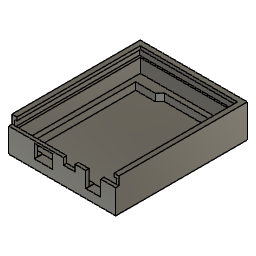
boitier VF Soufiani_Younousse (Autodesk Fusion 360 design; units mm, degrees)
Autodesk Fusion 360 part; units mm, degrees
note: some values were not read from the file. Set by a fixed rule: which sketch regions a step uses.
sketch "Esquisse1" plane through (0, 0, 0) normal (0, 0, 1) x (1, 0, 0)
  line L0 (0, 0) -> (53.1, 0)
  line L1 (53.1, 0) -> (53.1, 66.2)
  line L2 (0, 66.2) -> (0, 0)
  line L3 (40.9, 0) -> (49.9, 0)
  line L4 (49.9, 0) -> (49.9, -5.2)
  line L5 (49.9, -5.2) -> (40.9, -5.2)
  line L6 (40.9, -5.2) -> (40.9, 0)
  line L7 (11.5, 0) -> (18.8, 0)
  line L8 (18.8, 0) -> (18.8, -1.2)
  line L9 (18.8, -1.2) -> (11.5, -1.2)
  line L10 (11.5, -1.2) -> (11.5, 0)
  line L11 (53.1, 66.2) -> (50.8, 66.2) construction
  line L12 (50.8, 66.2) -> (48.7068, 69)
  line L13 (48.7068, 69) -> (14.6068, 69)
  line L14 (12.1, 66.2) -> (14.6068, 69)
  line L15 (53.1, 66.2) -> (50.8, 66.2)
  line L16 (12.1, 66.2) -> (0, 66.2)
  line L17 (40.9, 0) -> (49.9, 0)
  line L18 (11.5, 0) -> (18.8, 0)
  line L19 (0, 33.1) -> (53.1, 33.1) construction
  line L20 (26.55, 0) -> (26.55, 33.1) construction
  line L21 (0, 66.2) -> (0, 68.7) construction
  line L22 (0, 68.7) -> (53.1, 68.7) construction
  line L23 (53.1, 68.7) -> (53.1, 66.2) construction
  line L24 (-3, 72) -> (56.1, 72)
  line L25 (56.1, 72) -> (56.1, -3)
  line L26 (56.1, -3) -> (-3, -3)
  line L27 (-3, -3) -> (-3, 72)
  line L28 (-6, 75) -> (59.1, 75)
  line L29 (59.1, 75) -> (59.1, -5)
  line L30 (59.1, -5) -> (-6, -5)
  line L31 (-6, -5) -> (-6, 75)
  line L32 (26.55, 75) -> (26.55, -5) construction
  line L33 (11.5, -1.2) -> (11.5, -5)
  line L34 (18.8, -1.2) -> (18.8, -5)
  line L35 (15.15, 0) -> (15.15, -5) construction
  line L36 (9.55, 0) -> (20.75, 0)
  line L37 (20.75, 0) -> (20.75, -5)
  line L38 (20.75, -5) -> (9.55, -5)
  line L39 (9.55, -5) -> (9.55, 0)
  line L40 (15.15, 0) -> (15.15, -5) construction
  line L41 (-3, -3) -> (-6, -3)
  line L42 (56.1, -3) -> (59.1, -3)
  dimension "d1" = 66.2
  dimension "d13" = 53.1
  dimension "d14" = 3.2
  dimension "d15" = 9
  dimension "d16" = 5.2
  dimension "d17" = 11.5
  dimension "d18" = 7.3
  dimension "d19" = 1.2
  dimension "d21" = 2.3
  dimension "d22" = 38.7
  dimension "d25" = 34.1
  dimension "d43" = 3
  dimension "d44" = 3
  dimension "d45" = 3
  dimension "d46" = 3
  dimension "d47" = 3
  dimension "d48" = 3
  dimension "d52" = 11.2
  constraint horizontal L0
  constraint vertical L1
  constraint horizontal L15
  constraint vertical L2
  constraint coincident L0.start L2.end
  constraint horizontal L3
  constraint vertical L4
  constraint horizontal L5
  constraint vertical L6
  constraint coincident L0 L3.start
  constraint horizontal L7
  constraint vertical L8
  constraint horizontal L9
  constraint vertical L10
  constraint coincident L0 L7.start
  constraint perpendicular L1 L11
  constraint collinear L15 L16
  constraint horizontal L17
  constraint horizontal L18
  constraint midpoint L2 L19.start
  constraint midpoint L1 L19.end
  constraint midpoint L0 L20.start
  constraint midpoint L19 L20.end
  constraint perpendicular L13 L21
  constraint perpendicular L1 L22
  constraint perpendicular L15 L23
  constraint horizontal L24
  constraint vertical L25
  constraint horizontal L26
  constraint vertical L27
  constraint horizontal L28
  constraint vertical L29
  constraint horizontal L30
  constraint vertical L31
  constraint midpoint L28 L32.start
  constraint midpoint L30 L32.end
  constraint collinear L20 L32
  constraint coincident L30 L33.end
  constraint perpendicular L30 L33
  constraint coincident L30 L34.end
  constraint perpendicular L30 L34
  constraint midpoint L7 L35.start
  constraint coincident L30 L35.end
  constraint perpendicular L30 L35
  constraint horizontal L36
  constraint vertical L37
  constraint horizontal L38
  constraint vertical L39
  constraint coincident L30 L37.end
  constraint coincident L0 L36.start
  constraint midpoint L36 L35.start
  constraint midpoint L38 L35.end
  constraint collinear L35 L40
  constraint coincident L31 L41.end
  constraint perpendicular L31 L41
  constraint coincident L29 L42.end
  constraint perpendicular L29 L42
  measures "d1" distance of L0.start L2.start
  measures "d13" distance of L1.end L2.start
  measures "d14" distance of L1 L4
  measures "d15" distance of L4.end L5.end
  measures "d16" distance of L3.start L5.end
  measures "d17" distance of L2 L10
  measures "d18" distance of L8.end L9.end
  measures "d19" distance of L7.end L8.end
  measures "d21" distance of L1.end L11.end
  measures "d22" distance of L11.end L14.start
  measures "d25" distance of L12.end L13.end
  measures "d43" distance of L13 L24
  measures "d44" distance of L0 L26
  measures "d45" distance of L1 L25
  measures "d46" distance of L2 L27
  measures "d47" distance of L27 L31
  measures "d48" distance of L24 L28
  measures "d52" distance of L37 L39
extrude "Extrusion6" add sketch "Esquisse1" along normal blind 1 contours L0 L1 L2 L3 L7 L12 L13 L14 L15 L16 L17 L18 L36
extrude "Extrusion7" add sketch "Esquisse1" along normal blind 5.5 draft 1 contours L0 L1 L2 L4 L12 L13 L14 L15 L16 L24 L25 L26 L27 L39 | L0 L6 L26 L37
extrude "Extrusion8" add sketch "Esquisse1" along normal blind 20 contours L24 L25 L27 L28 L29 L31 L41 L42
extrude "Extrusion9" add sketch "Esquisse1" along normal blind 4.5 contours L0 L10 L26 L33 L36 L39 | L0 L7 L8 L9 L10 L18 L36 | L26 L30 L33 L38 L39 | L0 L8 L26 L34 L36 L37 | L9 L26 L33 L34 | L26 L30 L33 L34 L38 | L26 L30 L34 L37 L38 | L0 L3 L4 L6 L17 L26 | L4 L6 L26 L30
extrude "Extrusion10" add sketch "Esquisse1" along normal blind 14.8 contours L26 L30 L31 L39 L41 | L6 L26 L30 L37 | L4 L26 L29 L30 L42
sketch "Esquisse2" plane through (-3, 0, 0) normal (1, 0, 0) x (0, 1, 0)
  line L0 (-3, 5.5) -> (72, 5.5)
  line L1 (72, 5.5) -> (72, 20)
  line L2 (72, 20) -> (-3, 20)
  line L3 (-3, 20) -> (-3, 14.8)
  line L4 (-3, 14.8) -> (-3, 5.5)
  line L5 (-3, 20) -> (75, 20) construction
  line L6 (-3, 18) -> (72.5, 18)
  line L7 (72.5, 18) -> (72.5, 13.8)
  line L8 (72.5, 13.8) -> (-3, 13.8)
  line L9 (-3, 13.8) -> (-3, 18)
  dimension "d65" = 2
  dimension "d66" = 4.2
  dimension "d67" = 75.5
  constraint coincident L2.end L3.start
  constraint perpendicular L3 L5
  constraint horizontal L6
  constraint vertical L7
  constraint horizontal L8
  constraint vertical L9
  constraint coincident L3 L6.start
  measures "d65" distance of L5 L6
  measures "d66" distance of L6.end L7.end
  measures "d67" distance of L7.end L8.end
extrude "Extrusion11" cut sketch "Esquisse2" against normal blind 1.5 contours L1 L3 L4 L6 L8 L9
sketch "Esquisse3" plane through (56.1, 0, 0) normal (-1, 0, 0) x (0, -1, 0)
  line L0 (-72, 5.5) -> (3, 5.5)
  line L1 (3, 5.5) -> (3, 14.8)
  line L2 (3, 14.8) -> (3, 20)
  line L3 (3, 20) -> (-72, 20)
  line L4 (-72, 20) -> (-72, 5.5)
  line L5 (-72, 20) -> (3, 20) construction
  line L6 (-72, 18) -> (3, 18)
  line L7 (3, 18) -> (3, 13.8)
  line L8 (3, 13.8) -> (-72, 13.8)
  line L9 (-72, 13.8) -> (-72, 18)
  dimension "d70" = 4.2
  dimension "d71" = 2
  constraint coincident L3.end L4.start
  constraint coincident L2.end L3.start
  constraint horizontal L6
  constraint vertical L7
  constraint horizontal L8
  constraint vertical L9
  constraint coincident L2 L7.end
  constraint coincident L4 L6.start
  measures "d70" distance of L6.start L8.end
  measures "d71" distance of L5 L6
extrude "Extrusion12" cut sketch "Esquisse3" against normal blind 1.5 contours L1 L2 L4 L6 L7 L8 L9
sketch "Esquisse4" plane through (0, 72, 0) normal (0, -1, 0) x (1, 0, 0)
  line L0 (-3, 5.5) -> (56.1, 5.5)
  line L1 (56.1, 5.5) -> (56.1, 13.8)
  line L2 (56.1, 13.8) -> (57.6, 13.8)
  line L3 (57.6, 13.8) -> (57.6, 18)
  line L4 (57.6, 18) -> (56.1, 18)
  line L5 (56.1, 18) -> (56.1, 20)
  line L6 (56.1, 20) -> (-3, 20)
  line L7 (-3, 20) -> (-3, 18)
  line L8 (-3, 18) -> (-4.5, 18)
  line L9 (-4.5, 18) -> (-4.5, 13.8)
  line L10 (-4.5, 13.8) -> (-3, 13.8)
  line L11 (-3, 13.8) -> (-3, 5.5)
  line L12 (-4.5, 18) -> (57.6, 18)
  line L13 (57.6, 18) -> (57.6, 13.8)
  line L14 (57.6, 13.8) -> (-4.5, 13.8)
  line L15 (-4.5, 13.8) -> (-4.5, 18)
  constraint horizontal L12
  constraint vertical L13
  constraint horizontal L14
  constraint vertical L15
  constraint coincident L2.end L3.start
  constraint coincident L8.end L9.start
extrude "Extrusion13" add 2 faces at (43.9262, -1.0262, 4.5) (16.9905, -1.0262, 4.5) along direction (0, 0, 1) blind 0.8
sketch "Esquisse5" plane through (0, -3, 0) normal (0, 1, 0) x (-1, 0, 0)
  line L0 (-40.9, 5.5) -> (-20.75, 5.5)
  line L1 (-20.75, 5.5) -> (-20.75, 14.8)
  line L2 (-20.75, 14.8) -> (-40.9, 14.8)
  line L3 (-40.9, 14.8) -> (-40.9, 5.5)
  line L4 (-59.8312, 14.8) -> (5.1812, 14.8) construction
  line L5 (-50, 16) -> (-40.9, 16) construction
  line L6 (-20.75, 13.5) -> (-9.5, 13.5) construction
  line L7 (-40.9, 5.5) -> (-51, 5.5) construction
  line L8 (-51, 5.5) -> (-20.75, 5.5) construction
  line L9 (-9.284, 5.5) -> (-20.75, 5.5) construction
  line L10 (-50, 16) -> (-40.9, 16)
  line L11 (-40.9, 16) -> (-40.9, 14.8)
  line L12 (-40.9, 14.8) -> (-50, 14.8)
  line L13 (-50, 14.8) -> (-50, 16)
  line L14 (-20.75, 14.8) -> (-9.5, 14.8)
  line L15 (-9.5, 14.8) -> (-9.5, 13.5)
  line L16 (-9.5, 13.5) -> (-20.75, 13.5)
  line L17 (-20.75, 13.5) -> (-20.75, 14.8)
  line L18 (-27.325, 14.8) -> (-34.325, 14.8)
  line L19 (-34.325, 14.8) -> (-34.325, 10.8)
  line L20 (-34.325, 10.8) -> (-27.325, 10.8)
  line L21 (-27.325, 10.8) -> (-27.325, 14.8)
  line L22 (-20.75, 14.8) -> (-40.9, 14.8) construction
  line L23 (-40.9, 14.8) -> (-40.9, 5.5) construction
  line L24 (-40.9, 5.5) -> (-20.75, 5.5) construction
  line L25 (-20.75, 5.5) -> (-20.75, 14.8) construction
  line L26 (-30.825, 14.8) -> (-30.825, 10.8) construction
  line L27 (-30.825, 14.8) -> (-30.825, 5.5) construction
  dimension "d76" = 10.5
  dimension "d78" = 8
  dimension "d81" = 7
  dimension "d82" = 4
  constraint perpendicular L1 L4
  constraint coincident L3 L5.end
  constraint perpendicular L3 L5
  constraint coincident L1 L6.start
  constraint perpendicular L1 L6
  constraint coincident L0.start L3.end
  constraint perpendicular L3 L7
  constraint coincident L0.end L1.start
  constraint perpendicular L1 L8
  constraint perpendicular L1 L9
  constraint horizontal L10
  constraint vertical L11
  constraint horizontal L12
  constraint vertical L13
  constraint coincident L2.end L3.start
  constraint horizontal L14
  constraint vertical L15
  constraint horizontal L16
  constraint vertical L17
  constraint coincident L1.end L2.start
  constraint horizontal L18
  constraint vertical L19
  constraint horizontal L20
  constraint vertical L21
  constraint midpoint L4 L18.start
  constraint horizontal L22
  constraint vertical L23
  constraint horizontal L24
  constraint vertical L25
  constraint midpoint L18 L26.start
  constraint midpoint L20 L26.end
  constraint midpoint L22 L26.start
  constraint midpoint L24 L27.end
  constraint collinear L26 L27
  measures "d76" distance of L5 L7
  measures "d78" distance of L6 L9
  measures "d81" distance of L18.start L18.end
  measures "d82" distance of L18.start L20.end
extrude "Extrusion14" add sketch "Esquisse5" against normal blind 2 contours L10 L11 L12 L13 | L1 L14 L15 L16 L17
extrude "Extrusion16" cut sketch "Esquisse5" against normal blind 2 contours L2 L18 L19 L20 L21
extrude "Extrusion17" cut sketch "Esquisse4" against normal blind 1 contours L2 L3 L4 L8 L9 L10 L12 L13 L14 L15
extrude "Extrusion19" cut 1 faces at (46.9667, -3.6667, 16) along direction (0, 0, -1) blind 3
equation "d1 = longc1"
equation "longc1 = 66.2 mm" comment "longueur Carte"
equation "largc1 = 53.1 mm" comment "largueur Carte"
equation "diffdepH = 2.5 mm" comment "différence de hauteur entre la carte et la foorme du dessus"
equation "epchar = 11 mm" comment "épaisseur de l'entrée chargeur"
equation "depconn = 1.2 mm" comment "dépassement due a l'entrée usb-c"
equation "depchar = 5.2 mm" comment "dépassement du à l'entrée charqeur"
equation "larchar = 9 mm" comment "largeur de l'entrée chargeur"
equation "larconn = 7.3 mm" comment "largeur de l'entrée USB-C"
equation "distborconn = 11.5 mm" comment "distance entre l'entrée USB-C et le bord le plus proche"
equation "distborchar = 3.2 mm" comment "distance entre l'entrée chargeur et le bord le plus proche"
equation "diffdepD = 2.3 mm" comment "distance entre bordure droit  et le dépassement"
equation "d13 = largc1"
equation "d14 = distborchar"
equation "d15 = larchar"
equation "d16 = depchar"
equation "d17 = distborconn"
equation "d18 = larconn"
equation "d19 = depconn"
equation "largdep = 34.2 mm" comment "largeur du dépassement"
equation "d21 = diffdepD"
equation "epC = 4.5 mm" comment "épaisseur de la carte"
equation "epconn = 2.5 mm" comment "epaisseur entrée usb-c"
equation "diffCB = 3 mm" comment "espace entre bordure et carte"
equation "d43 = diffCB"
equation "d44 = diffCB"
equation "d45 = diffCB"
equation "d46 = diffCB"
equation "d47 = epB"
equation "d48 = epB"
equation "epB = 3 mm" comment "épaisseur de la boite"
equation "Lpu = 11.2 mm" comment "largeur de l'embout USB-c"
equation "Hpu = 8 mm" comment "Hauteur de l'embout USB-c"
equation "d52 = Lpu"
equation "d55 = 1 mm + epC"
equation "HB = 20 mm" comment "Hauteur Boite"
equation "epV = 3.2 mm" comment "épaisseur vitre"
equation "d59 = HB"
equation "d61 = epC"
equation "d63 = HB - 2 mm - epV"
equation "d66 = epV + 1 mm"
equation "d67 = 78.000001 mm - 2.5 mm"
equation "d70 = epV + 1 mm"
equation "d76 = HC"
equation "HC = 10.5 mm" comment "hauteur del'embout chargeur"
equation "d78 = Hpu"
equation "longpin = 3 mm"
